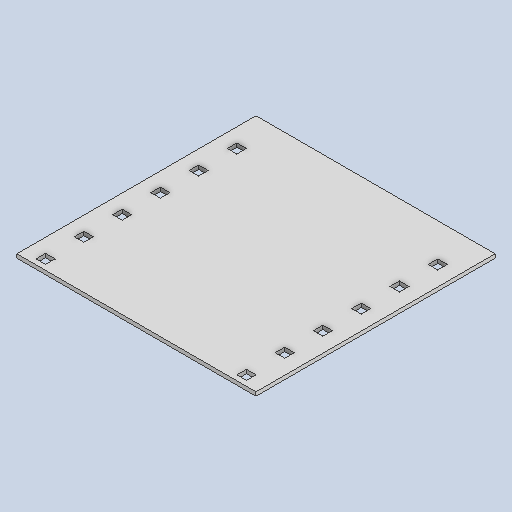
# Autodesk Inventor part: Платформа подъёмника
Saved by Autodesk Inventor 2023.2 (Build 272271030, 271C)
## iProperties
Created: 2025-03-18
Part Number: Платформа подъёмника
Material: Типовые
Document SubType Name: Modeling
Designer: Коноваленко
Density: 1 g/cm^3
Appearance: По умолчанию
Mass: 354.697 g
Surface Area: 1845.71 cm^2
Volume: 354.697 cm^3
Author: Коноваленко
Autodesk Inventor part; units mm, degrees
ref_plane "YZ Plane" through (0, 0, 0) normal (1, 0, 0) x (0, 1, 0)
ref_plane "XZ Plane" through (0, 0, 0) normal (0, 1, 0) x (-1, 0, 0)
ref_plane "XY Plane" through (0, 0, 0) normal (0, 0, 1) x (1, 0, 0)
sketch "Эскиз1" plane through (0, 0, 0) normal (0, 1, 0) x (-1, 0, 0)
  line L0 (125, 125) -> (-125, 125)
  line L1 (-125, 125) -> (-125, -125)
  line L2 (-125, -125) -> (125, -125)
  line L3 (125, -125) -> (125, 125)
  line L4 (125, 125) -> (-125, -125) construction
  line L5 (-125, 125) -> (125, -125) construction
  point P0 (0, 0)
  dimension "d0" = 250
  dimension "d1" = 250
  constraints: 12 end point, 2 midpoint, 2 parallel, 1 horizontal, 1 perpendicular
  measures "d0" distance of L1.end L2.end
  measures "d1" distance of L0.end L1.end
extrude "Выдавливание1" add sketch "Эскиз1" along normal blind 4
sketch "Эскиз2" plane through (0, 0, 0) normal (0, -1, 0) x (1, 0, 0)
  line L0 (-110.387511, 109.588885) -> (-110.387511, 119.588885)
  line L1 (-100.387511, 109.588885) -> (-110.387511, 109.588885)
  line L2 (-100.387511, 119.588885) -> (-100.387511, 109.588885)
  line L3 (-110.387511, 119.588885) -> (-100.387511, 119.588885)
  line L4 (-110.387511, 29.588885) -> (-110.387511, 39.588885)
  line L5 (-100.387511, 29.588885) -> (-110.387511, 29.588885)
  line L6 (-100.387511, 39.588885) -> (-100.387511, 29.588885)
  line L7 (-110.387511, 39.588885) -> (-100.387511, 39.588885)
  line L8 (-110.387511, -10.411115) -> (-110.387511, -0.411115)
  line L9 (-100.387511, -10.411115) -> (-110.387511, -10.411115)
  line L10 (-100.387511, -0.411115) -> (-100.387511, -10.411115)
  line L11 (-110.387511, -0.411115) -> (-100.387511, -0.411115)
  line L12 (125, 125) -> (125, -125)
  line L13 (-125, 125) -> (125, 125)
  line L14 (-125, -125) -> (-125, 125)
  line L15 (125, -125) -> (-125, -125)
  line L16 (109.612489, 109.588885) -> (109.612489, 119.588885)
  line L17 (109.612489, 119.588885) -> (99.612489, 119.588885)
  line L18 (99.612489, 119.588885) -> (99.612489, 109.588885)
  line L19 (99.612489, 109.588885) -> (109.612489, 109.588885)
  line L20 (109.612489, 29.588885) -> (109.612489, 39.588885)
  line L21 (109.612489, 39.588885) -> (99.612489, 39.588885)
  line L22 (99.612489, 39.588885) -> (99.612489, 29.588885)
  line L23 (99.612489, 29.588885) -> (109.612489, 29.588885)
  line L24 (109.612489, -10.411115) -> (109.612489, -0.411115)
  line L25 (109.612489, -0.411115) -> (99.612489, -0.411115)
  line L26 (99.612489, -0.411115) -> (99.612489, -10.411115)
  line L27 (99.612489, -10.411115) -> (109.612489, -10.411115)
  line L28 (109.612488, -50.411115) -> (109.612488, -40.411115)
  line L29 (109.612488, -40.411115) -> (99.612488, -40.411115)
  line L30 (99.612488, -40.411115) -> (99.612488, -50.411115)
  line L31 (99.612488, -50.411115) -> (109.612488, -50.411115)
  line L32 (109.612488, -90.411115) -> (109.612488, -80.411115)
  line L33 (109.612488, -80.411115) -> (99.612488, -80.411115)
  line L34 (99.612488, -80.411115) -> (99.612488, -90.411115)
  line L35 (99.612488, -90.411115) -> (109.612488, -90.411115)
  line L36 (-100.387512, -80.411115) -> (-100.387512, -90.411115)
  line L37 (-110.387512, -81.025031) -> (-100.387512, -81.025031)
  line L38 (-110.387512, -90.411115) -> (-110.387512, -80.411115)
  line L39 (-100.387512, -110) -> (-110.387512, -110)
  line L40 (-100.387512, -40.411115) -> (-100.387512, -50.411115)
  line L41 (-100.387512, -50.411115) -> (-110.387512, -50.411115)
  line L42 (-110.387512, -50.411115) -> (-110.387512, -40.411115)
  line L43 (-110.387512, -40.411115) -> (-100.387512, -40.411115)
  line L44 (-100.387512, 74.588885) -> (-100.387512, 69.588885)
  line L45 (-100.387512, 79.588885) -> (-100.387512, 74.588885)
  line L46 (-110.387512, 79.588885) -> (-100.387512, 79.588885)
  line L47 (-110.387512, 74.588885) -> (-110.387512, 79.588885)
  line L48 (-110.387512, 69.588885) -> (-110.387512, 74.588885)
  line L49 (-100.387512, 69.588885) -> (-110.387512, 69.588885)
  line L50 (109.612488, 79.588885) -> (99.612488, 79.588885)
  line L51 (99.612488, 69.588885) -> (109.612488, 69.588885)
  line L52 (99.612488, 74.588885) -> (99.612488, 69.588885)
  line L53 (109.612488, 69.588885) -> (109.612488, 74.588885)
  line L54 (109.612488, 74.588885) -> (109.612488, 79.588885)
  line L55 (99.612488, 79.588885) -> (99.612488, 74.588885)
  circle A0 centre (104.612488, -65.411115) radius 2
  circle A1 centre (104.612488, -25.411115) radius 2
  circle A2 centre (104.612488, 14.588885) radius 2
  circle A3 centre (104.612488, 54.588885) radius 2
  circle A4 centre (104.612488, 94.588885) radius 2
  circle A5 centre (-105.387512, 94.588885) radius 2
  circle A6 centre (-105.387512, 54.588885) radius 2
  circle A7 centre (-105.387512, 14.588885) radius 2
  circle A8 centre (-105.387512, -25.411115) radius 2
  circle A9 centre (-105.387512, -65.411115) radius 2
  point P0 (0, 0)
  constraints: 1 horizontal alignment
sketch "Эскиз2 outline for Выдавливание2" plane through (0, 0, 0) normal (0, -1, 0) x (1, 0, 0)
  line L0 (-110.387511, -10.411115) -> (-100.387511, -10.411115)
  line L1 (-110.387511, -0.411115) -> (-110.387511, -10.411115)
  line L2 (-100.387511, -0.411115) -> (-110.387511, -0.411115)
  line L3 (-100.387511, -10.411115) -> (-100.387511, -0.411115)
  line L4 (-110.387511, 29.588885) -> (-100.387511, 29.588885)
  line L5 (-110.387511, 39.588885) -> (-110.387511, 29.588885)
  line L6 (-100.387511, 39.588885) -> (-110.387511, 39.588885)
  line L7 (-100.387511, 29.588885) -> (-100.387511, 39.588885)
  line L8 (-110.387511, 109.588885) -> (-100.387511, 109.588885)
  line L9 (-110.387511, 119.588885) -> (-110.387511, 109.588885)
  line L10 (-100.387511, 119.588885) -> (-110.387511, 119.588885)
  line L11 (-100.387511, 109.588885) -> (-100.387511, 119.588885)
  line L12 (109.612488, -90.411115) -> (109.612488, -80.411115)
  line L13 (99.612488, -90.411115) -> (109.612488, -90.411115)
  line L14 (99.612488, -80.411115) -> (99.612488, -90.411115)
  line L15 (109.612488, -80.411115) -> (99.612488, -80.411115)
  line L16 (109.612488, -50.411115) -> (109.612488, -40.411115)
  line L17 (99.612488, -50.411115) -> (109.612488, -50.411115)
  line L18 (99.612488, -40.411115) -> (99.612488, -50.411115)
  line L19 (109.612488, -40.411115) -> (99.612488, -40.411115)
  line L20 (109.612489, -10.411115) -> (109.612489, -0.411115)
  line L21 (99.612489, -10.411115) -> (109.612489, -10.411115)
  line L22 (99.612489, -0.411115) -> (99.612489, -10.411115)
  line L23 (109.612489, -0.411115) -> (99.612489, -0.411115)
  line L24 (109.612489, 29.588885) -> (109.612489, 39.588885)
  line L25 (99.612489, 29.588885) -> (109.612489, 29.588885)
  line L26 (99.612489, 39.588885) -> (99.612489, 29.588885)
  line L27 (109.612489, 39.588885) -> (99.612489, 39.588885)
  line L28 (109.612489, 109.588885) -> (109.612489, 119.588885)
  line L29 (99.612489, 109.588885) -> (109.612489, 109.588885)
  line L30 (99.612489, 119.588885) -> (99.612489, 109.588885)
  line L31 (109.612489, 119.588885) -> (99.612489, 119.588885)
  line L32 (-100.387512, -80.411115) -> (-110.387512, -80.411115)
  line L33 (-100.387512, -90.411115) -> (-100.387512, -80.411115)
  line L34 (-110.387512, -90.411115) -> (-100.387512, -90.411115)
  line L35 (-110.387512, -80.411115) -> (-110.387512, -90.411115)
  line L36 (-100.387512, -40.411115) -> (-110.387512, -40.411115)
  line L37 (-100.387512, -50.411115) -> (-100.387512, -40.411115)
  line L38 (-110.387512, -50.411115) -> (-100.387512, -50.411115)
  line L39 (-110.387512, -40.411115) -> (-110.387512, -50.411115)
  line L40 (-100.387512, 69.588885) -> (-100.387512, 79.588885)
  line L41 (-100.387512, 79.588885) -> (-110.387512, 79.588885)
  line L42 (-110.387512, 79.588885) -> (-110.387512, 69.588885)
  line L43 (-110.387512, 69.588885) -> (-100.387512, 69.588885)
  line L44 (109.612488, 79.588885) -> (99.612488, 79.588885)
  line L45 (99.612488, 79.588885) -> (99.612488, 69.588885)
  line L46 (99.612488, 69.588885) -> (109.612488, 69.588885)
  line L47 (109.612488, 69.588885) -> (109.612488, 79.588885)
extrude "Выдавливание2" cut sketch "Эскиз2 outline for Выдавливание2" against normal up to surface (4 mm away)
